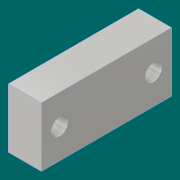
# Autodesk Inventor part: suppourtBlock
Saved by Autodesk Inventor 2016 (Build 200138000, 138)
## iProperties
Created: 2016-02-18
Part Number: suppourtBlock
Material: Aluminum 6061
Document SubType Name: Modeling
Designer: Sawaiz
Density: 2.7 g/cm^3
Appearance: Aluminum - Flat
Author: Sawaiz
Autodesk Inventor part; units mm, degrees
note: some values were not read from the file. Left out: dimensions or parameters whose unit could not be read.
ref_plane "YZ Plane" through (0, 0, 0) normal (1, 0, 0) x (0, 1, 0)
ref_plane "XZ Plane" through (0, 0, 0) normal (0, 1, 0) x (-1, 0, 0)
ref_plane "XY Plane" through (0, 0, 0) normal (0, 0, 1) x (1, 0, 0)
sketch "Sketch4" plane through (0, 0, 0) normal (0, 1, 0) x (-1, 0, 0)
  line L0 (-12.5, -5.708) -> (12.5, -5.708)
  line L1 (12.5, -5.708) -> (12.5, 5.708)
  line L2 (12.5, 5.708) -> (-12.5, 5.708)
  line L3 (-12.5, 5.708) -> (-12.5, -5.708)
  line L4 (-12.5, -5.708) -> (12.5, 5.708) construction
  line L5 (12.5, -5.708) -> (-12.5, 5.708) construction
  point P0 (0, 0)
  dimension "d22" = 11.416
  dimension "d23" = 25
  constraints: 12 end point, 2 midpoint, 2 parallel, 1 horizontal, 1 perpendicular
  measures "d22" distance of L0.end L1.end
  measures "d23" distance of L0.start L0.end
extrude "Extrusion3" add sketch "Sketch4" along normal mid plane 6.35
sketch "Sketch5" plane through (0, 3.175, 0) normal (0, 1, 0) x (1, 0, 0)
  line L0 (12.5, 5.708) -> (-12.5, 5.708) projected
  line L1 (-12.5, 5.708) -> (-12.5, -5.708) projected
  line L2 (-12.5, -5.708) -> (12.5, -5.708) projected
  line L3 (12.5, -5.708) -> (12.5, 5.708) projected
  line L4 (9, 0) -> (0, 0)
  dimension "d26" = 9
  constraints: 2 end point, 1 coincident, 1 horizontal
  measures "d26" distance of L4.start L4.end
hole "Hole2" at (9, 3.175, 0) direction (0, -1, 0) diameter 3.264 end through all clearance for "Socket Head Cap Screw" size "#4" standard "Ansi Unified Screw Threads"
mirror "Mirror2" about plane through (0, 0, 0) normal (1, 0, 0) of "Hole2"
equation "\"d22\" = 2 * silveringThickness + ScintillatorThickness + 2 * rubberizedCoating"
equation "\"d26\" = MountingScrewOffsett"
equation "\"OpticalFiberClearence\" = 0.071"
equation "\"ScintillatorEdgeClearence\" = 3"
equation "\"ShallowTrackDepth\" = 1.142"
equation "\"DeepTrackDepth\" = 5.571"
equation "\"FiberEdgeOffsett\" = 5"
equation "\"LoopLargeTrackRatio\" = 1.1"
equation "\"FiberSensorClerence\" = 0.5"
equation "\"MountingScrewOffsett\" = 9"
equation "\"silveringThickness\" = 0.2"
equation "\"mppcMountDepth\" = 6.35"
equation "\"ScintillatorThickness\" = 10"
body "Solid3"
